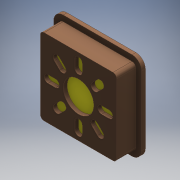
# Autodesk Inventor part: button1
Saved by Autodesk Inventor 2016 (Build 200138000, 138)
## iProperties
Created: 2017-11-06
Part Number: button1
Material: Bronze, Soft Tin
Document SubType Name: Modeling
Designer: Davide
Density: 8.874 g/cm^3
Appearance: Bronze - Satin
Author: Davide
Autodesk Inventor part; units mm, degrees
ref_plane "YZ Plane" through (0, 0, 0) normal (1, 0, 0) x (0, 1, 0)
ref_plane "XZ Plane" through (0, 0, 0) normal (0, 1, 0) x (-1, 0, 0)
ref_plane "XY Plane" through (0, 0, 0) normal (0, 0, 1) x (1, 0, 0)
sketch "Sketch1" plane through (0, 0, 0) normal (0, 1, 0) x (-1, 0, 0)
  line L0 (9, -10) -> (-9, -10)
  line L1 (-10, -9) -> (-10, 9)
  line L2 (-9, 10) -> (9, 10)
  line L3 (10, 9) -> (10, -9)
  line L4 (10, 10) -> (-10, -10) construction
  line L5 (10, -10) -> (-10, 10) construction
  arc A0 (10, 9) -> (9, 10) centre (9, 9) ccw
  arc A1 (9, -10) -> (10, -9) centre (9, -9) ccw
  arc A2 (-10, -9) -> (-9, -10) centre (-9, -9) ccw
  arc A3 (-9, 10) -> (-10, 9) centre (-9, 9) ccw
  point P0 (0, 0)
  point P1 (0, 0)
  dimension "d7" = 20
  dimension "d9" = 20
  dimension "d10" = 1
  constraints: 12 end point, 8 point on circle, 8 point on line, 8 tangent, 4 centre point, 3 equal radius, 2 parallel, 1 coincident, 1 horizontal, 1 midpoint, 1 perpendicular
  measures "d7" distance of L5.start L4.end
  measures "d9" distance of L4.end L5.end
  measures "d10" radius of A0
extrude "Extrusion1" add sketch "Sketch1" along normal blind 5
sketch "Sketch2" plane through (0, 5, 0) normal (0, 1, 0) x (1, 0, 0)
  line L0 (-10, 9) -> (-10, -9) projected
  arc A0 (-10, -9) -> (-9, -10) centre (-9, -9) ccw projected
  line L1 (-9, -10) -> (9, -10) projected
  arc A1 (9, -10) -> (10, -9) centre (9, -9) ccw projected
  line L2 (10, -9) -> (10, 9) projected
  arc A2 (10, 9) -> (9, 10) centre (9, 9) ccw projected
  line L3 (9, 10) -> (-9, 10) projected
  arc A3 (-9, 10) -> (-10, 9) centre (-9, 9) ccw projected
  line L4 (9, -11.5) -> (-9, -11.5)
  arc A4 (-11.5, -9) -> (-9, -11.5) centre (-9, -9) ccw
  line L5 (-11.5, -9) -> (-11.5, 9)
  arc A5 (-9, 11.5) -> (-11.5, 9) centre (-9, 9) ccw
  line L6 (-9, 11.5) -> (9, 11.5)
  arc A6 (11.5, 9) -> (9, 11.5) centre (9, 9) ccw
  line L7 (11.5, 9) -> (11.5, -9)
  arc A7 (9, -11.5) -> (11.5, -9) centre (9, -9) ccw
  circle A8 centre (0, 0) radius 2.75
  dimension "d16" = 1.5
  dimension "d19" = 5.5
  constraints: 8 end point, 8 point on circle, 5 centre point, 1 coincident, 7 other
  measures "d16" distance between parallel lines of L1 L4
  measures "d19" diameter of A8
extrude "Extrusion3" add sketch "Sketch2" along normal blind 1 contours A3 L3 A2 L2 A1 L1 A0 L0 | L4 A4 L5 A5 L6 A6 L7 A7
sketch "Sketch3" plane through (0, 0, 0) normal (0, -1, 0) x (1, 0, 0)
  circle A0 centre (0, 0) radius 4
  arc A1 (-6, -1) -> (-6, 1) centre (-6, 0) ccw
  arc A2 (-8, 1) -> (-8, -1) centre (-8, 0) ccw
  line L0 (-6, -1) -> (-8, -1)
  line L1 (-6, 1) -> (-8, 1)
  line L2 (0, 0) -> (-5, 0) construction
  arc A3 (-3.5355, -4.9497) -> (-4.9497, -3.5355) centre (-4.2426, -4.2426) ccw
  line L3 (-3.5355, -4.9497) -> (-4.9497, -6.364)
  line L4 (-4.9497, -3.5355) -> (-6.364, -4.9497)
  arc A4 (-6.364, -4.9497) -> (-4.9497, -6.364) centre (-5.6569, -5.6569) ccw
  arc A5 (1, -6) -> (-1, -6) centre (0, -6) ccw
  line L5 (1, -6) -> (1, -8)
  line L6 (-1, -6) -> (-1, -8)
  arc A6 (-1, -8) -> (1, -8) centre (0, -8) ccw
  arc A7 (4.9497, -3.5355) -> (3.5355, -4.9497) centre (4.2426, -4.2426) ccw
  line L7 (4.9497, -3.5355) -> (6.364, -4.9497)
  line L8 (3.5355, -4.9497) -> (4.9497, -6.364)
  arc A8 (4.9497, -6.364) -> (6.364, -4.9497) centre (5.6569, -5.6569) ccw
  arc A9 (6, 1) -> (6, -1) centre (6, 0) ccw
  line L9 (6, 1) -> (8, 1)
  line L10 (6, -1) -> (8, -1)
  arc A10 (8, -1) -> (8, 1) centre (8, 0) ccw
  arc A11 (3.5355, 4.9497) -> (4.9497, 3.5355) centre (4.2426, 4.2426) ccw
  line L11 (3.5355, 4.9497) -> (4.9497, 6.364)
  line L12 (4.9497, 3.5355) -> (6.364, 4.9497)
  arc A12 (6.364, 4.9497) -> (4.9497, 6.364) centre (5.6569, 5.6569) ccw
  arc A13 (-1, 6) -> (1, 6) centre (0, 6) ccw
  line L13 (-1, 6) -> (-1, 8)
  line L14 (1, 6) -> (1, 8)
  arc A14 (1, 8) -> (-1, 8) centre (0, 8) ccw
  arc A15 (-4.9497, 3.5355) -> (-3.5355, 4.9497) centre (-4.2426, 4.2426) ccw
  line L15 (-4.9497, 3.5355) -> (-6.364, 4.9497)
  line L16 (-3.5355, 4.9497) -> (-4.9497, 6.364)
  arc A16 (-4.9497, 6.364) -> (-6.364, 4.9497) centre (-5.6569, 5.6569) ccw
  dimension "d24" = 2
  dimension "d25" = 2
  dimension "d26" = 2
  dimension "d27" = 6
  dimension "d28" = 360
  dimension "d29" = 16
  dimension "d37" = 8
  constraints: 34 end point, 33 point on circle, 17 centre point, 3 coincident, 2 point on line, 2 tangent, 1 horizontal, 81 other
  measures "d24" diameter of A1
  measures "d25" diameter of A2
  measures "d26" distance of A2.centre A1.centre
  measures "d27" distance of A1.centre point (0, 0)
  measures "d29" distance of A2.centre A10.centre
  measures "d37" diameter of A0
extrude "Extrusion4" cut sketch "Sketch3" against normal blind 1
hole "Hole1" at (0, 5, 0) direction (0, -1, 0) diameter 5.5 depth 3
equation "\"d7\" = button_side"
equation "\"d9\" = d7"
equation "\"d24\" = d25"
equation "\"d25\" = d26"
equation "\"d27\" = 3 * d26"
equation "\"d37\" = 4 * d26"
equation "\"d0\" = 122"
equation "\"d1\" = 77"
equation "\"d4\" = 19"
equation "\"d5\" = 1"
equation "\"d8\" = 25"
equation "\"d13\" = 1.5"
equation "\"d14\" = 0"
equation "\"d15\" = 2"
equation "\"d30\" = 3.1"
equation "\"d31\" = 3"
equation "\"d33\" = 3"
equation "\"d34\" = 2"
equation "\"d36\" = 3"
equation "\"d38\" = 90deg"
equation "\"d39\" = 8"
equation "\"d40\" = 118deg"
equation "\"d44\" = 0"
equation "\"d45\" = 1.2"
equation "\"d46\" = 2"
equation "\"d47\" = 0"
equation "\"d50\" = 25"
equation "\"button_side\" = 20"
equation "\"d3\" = 1.01 * button_side"
equation "\"d2\" = d3"
body "Solid1"
